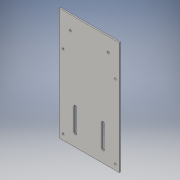
# Autodesk Inventor part: Part2
Saved by Autodesk Inventor 2016 (Build 200138000, 138)
## iProperties
Created: 2015-10-15
Part Number: Part2
Material: Generic
Document SubType Name: Modeling
Designer: hozhu
Density: 1 g/cm^3
Appearance: Default
Author: hozhu
Autodesk Inventor part; units mm, degrees
ref_plane "YZ Plane" through (0, 0, 0) normal (1, 0, 0) x (0, 1, 0)
ref_plane "XZ Plane" through (0, 0, 0) normal (0, 1, 0) x (-1, 0, 0)
ref_plane "XY Plane" through (0, 0, 0) normal (0, 0, 1) x (1, 0, 0)
sketch "Sketch1" plane through (0, 0, 0) normal (0, 0, 1) x (1, 0, 0)
  line L0 (-68.58, -128.7145) -> (68.58, -128.7145)
  line L1 (68.58, -128.7145) -> (68.58, 128.7145)
  line L2 (68.58, 128.7145) -> (-68.58, 128.7145)
  line L3 (-68.58, 128.7145) -> (-68.58, -128.7145)
  line L4 (-68.58, -128.7145) -> (68.58, 128.7145) construction
  line L5 (68.58, -128.7145) -> (-68.58, 128.7145) construction
  point P0 (0, 0)
  dimension "d0" = 137.16
  dimension "d1" = 257.429
  constraints: 12 end point, 2 midpoint, 2 parallel, 1 horizontal, 1 perpendicular
  measures "d0" distance of L1.end L2.end
  measures "d1" distance of L2.end L0.start
extrude "Extrusion1" add sketch "Sketch1" against normal blind 3.175
sketch "Sketch2" plane through (0, 0, 0) normal (0, 0, 1) x (1, 0, 0)
  circle A0 centre (-59.69, 52.5145) radius 2.0955
  line L0 (-68.58, 128.7145) -> (-68.58, -128.7145) projected
  line L1 (-68.58, 128.7145) -> (68.58, 128.7145) projected
  circle A1 centre (59.69, 52.5145) radius 2.0955
  line L2 (68.58, -128.7145) -> (68.58, 128.7145) projected
  circle A2 centre (-59.69, -116.0145) radius 2.0955
  circle A3 centre (59.69, -116.0145) radius 2.0955
  line L3 (-68.58, -128.7145) -> (68.58, -128.7145) projected
  point P0 (0, 0)
  dimension "d4" = 8.89
  dimension "d5" = 76.2
  dimension "d6" = 76.2
  dimension "d7" = 8.89
  dimension "d8" = 4.191
  dimension "d9" = 12.7
  dimension "d10" = 8.89
  dimension "d11" = 8.89
  dimension "d12" = 12.7
  dimension "d13" = 4.191
  dimension "d21" = 4.191
  dimension "d22" = 4.191
  constraints: 4 centre point
  measures "d4" distance from line of L0 A0.centre
  measures "d5" distance from line of L1 A0.centre
  measures "d6" distance from line of L1 A1.centre
  measures "d7" distance from line of A1.centre L2
  measures "d8" diameter of A1
  measures "d9" distance from line of L3 A2.centre
  measures "d10" distance from line of L0 A2.centre
  measures "d11" distance from line of L2 A3.centre
  measures "d12" distance from line of L3 A3.centre
  measures "d13" diameter of A0
  measures "d21" diameter of A2
  measures "d22" diameter of A3
hole "Hole1" at (-59.69, 52.5145, 0) at (59.69, 52.5145, 0) at (-59.69, -116.0145, 0) at (59.69, -116.0145, 0) direction (0, 0, -1) diameter 4.191 end through all
sketch "Sketch4" plane through (0, 0, 0) normal (0, 0, 1) x (1, 0, 0)
  line L0 (-35.179, -49.0855) -> (-35.179, -99.8855)
  line L1 (-28.321, -49.0855) -> (-28.321, -99.8855)
  line L2 (28.321, -49.0855) -> (28.321, -99.8855)
  line L3 (35.179, -49.0855) -> (35.179, -99.8855)
  line L4 (-68.58, 128.7145) -> (-68.58, -128.7145) projected
  line L5 (68.58, -128.7145) -> (68.58, 128.7145) projected
  line L6 (-68.58, -128.7145) -> (68.58, -128.7145) projected
  arc A0 (-28.321, -49.0855) -> (-35.179, -49.0855) centre (-31.75, -49.0855) ccw
  arc A1 (-35.179, -99.8855) -> (-28.321, -99.8855) centre (-31.75, -99.8855) ccw
  arc A2 (35.179, -49.0855) -> (28.321, -49.0855) centre (31.75, -49.0855) ccw
  arc A3 (28.321, -99.8855) -> (35.179, -99.8855) centre (31.75, -99.8855) ccw
  point P0 (0, 0)
  dimension "d23" = 6.858
  dimension "d24" = 6.858
  dimension "d25" = 33.401
  dimension "d26" = 50.8
  dimension "d27" = 33.401
  dimension "d28" = 28.829
  dimension "d29" = 28.829
  dimension "d30" = 28.829
  dimension "d31" = 28.829
  dimension "d32" = 50.8
  dimension "d33" = 50.8
  dimension "d34" = 50.8
  constraints: 8 end point, 8 point on circle, 4 centre point, 4 tangent, 4 vertical
  measures "d23" distance of L1.end L0.end
  measures "d24" distance between parallel lines of L3 L2
  measures "d25" distance between parallel lines of L4 L0
  measures "d26" distance of L3.start L3.end
  measures "d27" distance between parallel lines of L5 L3
  measures "d28" distance from line of L6 L0.end
  measures "d29" distance from line of L6 L1.end
  measures "d30" distance from line of L6 L2.end
  measures "d31" distance from line of L6 L3.end
  measures "d32" distance of L0.start L0.end
  measures "d33" distance of L1.start L1.end
  measures "d34" distance of L2.start L2.end
extrude "Extrusion2" cut sketch "Sketch4" against normal blind 3.175
sketch "Sketch5" plane through (0, 0, 0) normal (0, 0, 1) x (1, 0, 0)
  line L0 (-68.58, 128.7145) -> (68.58, 128.7145) projected
  line L1 (68.58, 128.7145) -> (68.58, -128.7145) projected
  point P0 (0, 0)
  point P1 (-43.3324, 96.9645)
  point P2 (43.3324, 96.9645)
  dimension "d37" = 31.75
  dimension "d38" = 86.6648
  dimension "d39" = 31.75
  dimension "d40" = 25.2476
  measures "d37" distance from line of L0 point (-43.332, 96.964)
  measures "d38" distance of point (-43.332, 96.964) point (43.332, 96.964)
  measures "d39" distance from line of L0 point (43.332, 96.964)
  measures "d40" distance from line of L1 point (43.332, 96.964)
hole "Hole2" at (-43.3324, 96.9645, 0) at (43.3324, 96.9645, 0) direction (0, 0, -1) diameter 4.4704 end through all
sketch "battery_buzzer" plane through (0, 0, 0) normal (0, 0, 1) x (1, 0, 0)
  line L0 (-50.8, 39.8145) -> (50.8, 39.8145)
  line L1 (50.8, 39.8145) -> (50.8, -36.3855)
  line L2 (50.8, -36.3855) -> (-50.8, -36.3855)
  line L3 (-50.8, -36.3855) -> (-50.8, 39.8145)
  line L4 (68.58, -128.7145) -> (68.58, 128.7145) projected
  line L5 (68.58, 128.7145) -> (-68.58, 128.7145) projected
  line L6 (-68.58, 128.7145) -> (-68.58, -128.7145) projected
  line L7 (-44.45, 33.4645) -> (-11.43, 33.4645)
  line L8 (-11.43, 33.4645) -> (-11.43, 5.5245)
  line L9 (-11.43, 5.5245) -> (-44.45, 5.5245)
  line L10 (-44.45, 5.5245) -> (-44.45, 33.4645)
  circle A0 centre (-40.64, 29.6545) radius 1.651
  circle A1 centre (-40.64, 8.6995) radius 1.651
  circle A2 centre (-15.24, 8.6995) radius 1.651
  line L11 (0.508, 33.4645) -> (33.528, 33.4645)
  line L12 (33.528, 33.4645) -> (33.528, 5.5245)
  line L13 (33.528, 5.5245) -> (0.508, 5.5245)
  line L14 (0.508, 5.5245) -> (0.508, 33.4645)
  circle A3 centre (4.318, 29.6545) radius 1.651
  circle A4 centre (4.318, 8.6995) radius 1.651
  circle A5 centre (29.718, 8.6995) radius 1.651
  line L15 (-44.45, 1.7145) -> (-11.43, 1.7145)
  line L16 (-11.43, 1.7145) -> (-11.43, -26.2255)
  line L17 (-11.43, -26.2255) -> (-44.45, -26.2255)
  line L18 (-44.45, -26.2255) -> (-44.45, 1.7145)
  circle A6 centre (-40.64, -2.0955) radius 1.651
  circle A7 centre (-40.64, -23.0505) radius 1.651
  circle A8 centre (-15.2413, -22.7965) radius 1.651
  line L19 (33.5293, 1.9685) -> (33.5293, -27.2717)
  circle A9 centre (29.718, -23.0505) radius 1.651
  line L20 (33.5293, -27.2717) -> (0.5093, -27.2717)
  line L21 (0.5093, 1.9685) -> (33.5293, 1.9685)
  circle A10 centre (4.3193, -22.7965) radius 1.651
  circle A11 centre (4.3193, -1.8415) radius 1.651
  line L22 (0.5093, -27.2717) -> (0.5093, 1.9685)
  point P0 (-1.6153, -4.4833)
  point P1 (48.3688, -4.4833)
  dimension "d48" = 17.78
  dimension "d49" = 88.9
  dimension "d50" = 76.2
  dimension "d51" = 17.78
  dimension "d52" = 33.02
  dimension "d54" = 3.302
  dimension "d55" = 3.302
  dimension "d57" = 3.81
  dimension "d58" = 3.81
  dimension "d59" = 3.81
  dimension "d60" = 20.955
  dimension "d62" = 25.4
  dimension "d74" = 33.02
  dimension "d75" = 3.302
  dimension "d76" = 3.302
  dimension "d77" = 3.81
  dimension "d78" = 3.81
  dimension "d79" = 3.81
  dimension "d80" = 20.955
  dimension "d81" = 25.4
  dimension "d183" = 6.35
  dimension "d184" = 6.35
  dimension "d185" = 6.35
  dimension "d186" = 27.94
  dimension "d205" = 80.518
  dimension "d206" = 33.02
  dimension "d207" = 3.302
  dimension "d208" = 3.302
  dimension "d209" = 3.81
  dimension "d210" = 3.81
  dimension "d211" = 3.81
  dimension "d212" = 20.955
  dimension "d213" = 25.4
  dimension "d214" = 33.02
  dimension "d215" = 3.302
  dimension "d216" = 3.302
  dimension "d217" = 3.81
  dimension "d218" = 3.81
  dimension "d219" = 3.81
  dimension "d220" = 20.955
  dimension "d221" = 25.4
  dimension "d222" = 27.94
  dimension "d223" = 41.656
  dimension "d225" = 80.518
  dimension "d227" = 6.35
  dimension "d230" = 62.865
  dimension "d231" = 62.865
  constraints: 40 end point, 13 perpendicular, 12 centre point, 5 horizontal, 2 parallel
  measures "d48" distance between parallel lines of L4 L1
  measures "d49" distance between parallel lines of L5 L0
  measures "d50" distance of L0.end L1.end
  measures "d51" distance between parallel lines of L6 L3
  measures "d52" distance of L7.start L7.end
  measures "d54" diameter of A0
  measures "d55" diameter of A1
  measures "d57" distance from line of L7 A0.centre
  measures "d58" distance from line of L10 A1.centre
  measures "d59" distance from line of L10 A0.centre
  measures "d60" distance of A1.centre A0.centre
  measures "d62" distance of A1.centre A2.centre
  measures "d74" distance of L11.start L12.start
  measures "d75" diameter of A3
  measures "d76" diameter of A4
  measures "d77" distance from line of L11 A3.centre
  measures "d78" distance from line of L14 A4.centre
  measures "d79" distance from line of L14 A3.centre
  measures "d80" distance of A4.centre A3.centre
  measures "d81" distance of A4.centre A5.centre
  measures "d183" distance between parallel lines of L3 L10
  measures "d184" distance between parallel lines of L0 L7
  measures "d185" distance between parallel lines of L0 L11
  measures "d186" distance of L7.end L8.end
  measures "d205" distance from line of L3 A5.centre
  measures "d206" distance of L15.start L15.end
  measures "d207" diameter of A6
  measures "d208" diameter of A7
  measures "d209" distance from line of L15 A6.centre
  measures "d210" distance from line of L18 A7.centre
  measures "d211" distance from line of L18 A6.centre
  measures "d212" distance of A7.centre A6.centre
  measures "d213" distance of A7.centre A8.centre
  measures "d214" distance of L21.start L19.start
  measures "d215" diameter of A11
  measures "d216" diameter of A10
  measures "d217" distance from line of L21 A11.centre
  measures "d218" distance from line of L22 A10.centre
  measures "d219" distance from line of L22 A11.centre
  measures "d220" distance of A10.centre A11.centre
  measures "d221" distance of A10.centre A9.centre
  measures "d222" distance of L15.end L17.start
  measures "d223" distance from line of L0 A11.centre
  measures "d225" distance from line of L3 A9.centre
  measures "d227" distance between parallel lines of L3 L18
  measures "d230" distance from line of A7.centre L0
  measures "d231" distance from line of L0 A9.centre
sketch "grizzly_bear" plane through (0, 0, 0) normal (0, 0, 1) x (1, 0, 0)
  line L0 (-50.8, 39.8145) -> (50.8, 39.8145)
  line L1 (50.8, 39.8145) -> (50.8, -36.3855)
  line L2 (50.8, -36.3855) -> (-50.8, -36.3855)
  line L3 (-50.8, -36.3855) -> (-50.8, 39.8145)
  line L4 (-68.58, 128.7145) -> (-68.58, -128.7145) projected
  line L5 (68.58, -128.7145) -> (68.58, 128.7145) projected
  line L6 (68.58, 128.7145) -> (-68.58, 128.7145) projected
  line L7 (-43.688, -8.4455) -> (32.512, -8.4455)
  line L8 (32.512, -8.4455) -> (32.512, 32.8295)
  line L9 (32.512, 32.8295) -> (-43.688, 32.8295)
  line L10 (-43.688, 32.8295) -> (-43.688, -8.4455)
  circle A0 centre (-40.64, 29.6545) radius 1.651
  circle A1 centre (29.718, -5.6515) radius 1.651
  circle A2 centre (29.718, 29.6545) radius 1.651
  circle A3 centre (21.123, -3.4255) radius 0.45
  circle A4 centre (16.723, -3.4255) radius 0.45
  dimension "d100" = 17.78
  dimension "d101" = 17.78
  dimension "d102" = 88.9
  dimension "d103" = 76.2
  dimension "d187" = 3.302
  dimension "d188" = 0.9
  dimension "d189" = 76.2
  dimension "d190" = 41.275
  dimension "d191" = 2.794
  dimension "d192" = 3.175
  dimension "d193" = 38.481
  dimension "d194" = 73.406
  dimension "d195" = 11.389
  dimension "d196" = 36.255
  dimension "d197" = 15.789
  dimension "d198" = 36.255
  dimension "d199" = 73.152
  dimension "d200" = 3.175
  dimension "d203" = 10.16
  dimension "d204" = 10.16
  constraints: 16 end point, 5 centre point, 3 equal radius, 3 parallel, 3 perpendicular, 1 horizontal
  measures "d100" distance between parallel lines of L4 L3
  measures "d101" distance between parallel lines of L5 L1
  measures "d102" distance between parallel lines of L6 L0
  measures "d103" distance of L0.end L1.end
  measures "d187" diameter of A2
  measures "d188" diameter of A3
  measures "d189" distance between parallel lines of L8 L10
  measures "d190" distance between parallel lines of L7 L9
  measures "d191" distance from line of A2.centre L8
  measures "d192" distance from line of A2.centre L9
  measures "d193" distance from line of A1.centre L9
  measures "d194" distance from line of A1.centre L10
  measures "d195" distance from line of A3.centre L8
  measures "d196" distance from line of A3.centre L9
  measures "d197" distance from line of A4.centre L8
  measures "d198" distance from line of A4.centre L9
  measures "d199" distance from line of A0.centre L8
  measures "d200" distance from line of A0.centre L9
  measures "d203" distance from line of L0 A0.centre
  measures "d204" distance from line of L3 A0.centre
sketch "Smartsensor" plane through (0, 0, 0) normal (0, 0, 1) x (1, 0, 0)
  line L0 (-34.6866, -23.8471) -> (-34.6866, 4.0929)
  line L1 (-34.6866, 4.0929) -> (-1.6666, 4.0929)
  line L2 (-1.6666, 4.0929) -> (-1.6666, -23.8471)
  line L3 (-34.6866, -23.8471) -> (-1.6666, -23.8471)
  circle A0 centre (-30.8766, 0.2829) radius 1.651
  circle A1 centre (-5.4766, -20.6721) radius 1.651
  circle A2 centre (-4.2066, -16.2271) radius 1
  circle A3 centre (-4.2066, -13.6871) radius 1
  circle A4 centre (-4.2066, -11.1471) radius 1
  circle A5 centre (-4.2066, -8.6071) radius 1
  circle A6 centre (-4.2066, -6.0671) radius 1
  circle A7 centre (-4.2066, -3.5271) radius 1
  line L4 (0.8734, -23.8471) -> (0.8734, 4.0929)
  line L5 (0.8734, 4.0929) -> (33.8934, 4.0929)
  line L6 (33.8934, 4.0929) -> (33.8934, -23.8471)
  line L7 (0.8734, -23.8471) -> (33.8934, -23.8471)
  circle A8 centre (4.6834, 0.2829) radius 1.651
  circle A9 centre (30.0834, -20.6721) radius 1.651
  circle A10 centre (31.3534, -16.2271) radius 1
  circle A11 centre (31.3534, -13.6871) radius 1
  circle A12 centre (31.3534, -11.1471) radius 1
  circle A13 centre (31.3534, -8.6071) radius 1
  circle A14 centre (31.3534, -6.0671) radius 1
  circle A15 centre (31.3534, -3.5271) radius 1
  line L8 (-50.8, 39.8145) -> (50.8, 39.8145)
  line L9 (50.8, 39.8145) -> (50.8, -36.3855)
  line L10 (50.8, -36.3855) -> (-50.8, -36.3855)
  line L11 (-50.8, -36.3855) -> (-50.8, 39.8145)
  line L12 (68.58, -128.7145) -> (68.58, 128.7145) projected
  line L13 (-68.58, 128.7145) -> (-68.58, -128.7145) projected
  line L14 (68.58, 128.7145) -> (-68.58, 128.7145) projected
  point P0 (0, 0)
  dimension "d104" = 17.78
  dimension "d105" = 17.78
  dimension "d106" = 88.9
  dimension "d107" = 76.2
  constraints: 24 end point, 16 centre point, 2 parallel, 1 horizontal, 1 perpendicular
  measures "d104" distance between parallel lines of L12 L9
  measures "d105" distance between parallel lines of L13 L11
  measures "d106" distance between parallel lines of L14 L8
  measures "d107" distance of L10.end L8.start
sketch "SmartsensorPowered" plane through (0, 0, 0) normal (0, 0, 1) x (1, 0, 0)
  line L0 (-31.115, 32.8295) -> (-3.175, 32.8295)
  line L1 (-3.175, 32.8295) -> (-3.175, -26.8605)
  line L2 (-3.175, -26.8605) -> (-31.115, -26.8605)
  line L3 (-31.115, -26.8605) -> (-31.115, 32.8295)
  circle A0 centre (-27.94, 29.6545) radius 1.651
  circle A1 centre (-27.305, -23.0505) radius 1.651
  circle A2 centre (-6.35, 2.3495) radius 1.651
  circle A3 centre (-6.35, 29.6545) radius 1.651
  circle A4 centre (18.415, -23.0505) radius 1.651
  circle A5 centre (39.37, 2.3495) radius 1.651
  circle A6 centre (17.78, 29.6545) radius 1.651
  line L4 (14.605, -26.8605) -> (14.605, 32.8295)
  circle A7 centre (39.37, 29.6545) radius 1.651
  line L5 (14.605, 32.8295) -> (42.545, 32.8295)
  line L6 (42.545, 32.8295) -> (42.545, -26.8605)
  line L7 (42.545, -26.8605) -> (14.605, -26.8605)
  line L8 (-50.8, 39.8145) -> (50.8, 39.8145)
  line L9 (50.8, 39.8145) -> (50.8, -36.3855)
  line L10 (50.8, -36.3855) -> (-50.8, -36.3855)
  line L11 (-50.8, -36.3855) -> (-50.8, 39.8145)
  line L12 (-68.58, 128.7145) -> (-68.58, -128.7145) projected
  line L13 (68.58, 128.7145) -> (68.58, -128.7145) projected
  line L14 (68.58, 128.7145) -> (-68.58, 128.7145) projected
  point P0 (0, 0)
  dimension "d108" = 27.94
  dimension "d109" = 59.69
  dimension "d110" = 3.175
  dimension "d111" = 3.175
  dimension "d112" = 3.302
  dimension "d113" = 3.302
  dimension "d114" = 3.175
  dimension "d115" = 3.175
  dimension "d116" = 3.81
  dimension "d117" = 3.81
  dimension "d118" = 3.302
  dimension "d119" = 30.48
  dimension "d120" = 3.175
  dimension "d121" = 3.302
  dimension "d122" = 27.94
  dimension "d123" = 59.69
  dimension "d124" = 3.175
  dimension "d125" = 3.175
  dimension "d126" = 3.302
  dimension "d127" = 3.302
  dimension "d128" = 3.175
  dimension "d129" = 3.175
  dimension "d130" = 3.81
  dimension "d131" = 3.81
  dimension "d132" = 3.302
  dimension "d133" = 30.48
  dimension "d134" = 3.175
  dimension "d135" = 3.302
  dimension "d136" = 17.78
  dimension "d137" = 17.78
  dimension "d138" = 17.78
  dimension "d139" = 88.9
  dimension "d140" = 76.2
  dimension "d228" = 10.16
  dimension "d229" = 22.86
  constraints: 24 end point, 8 centre point, 6 parallel, 3 horizontal, 3 perpendicular, 1 collinear
  measures "d108" distance of L0.start L0.end
  measures "d109" distance of L2.end L0.start
  measures "d110" distance from line of L3 A0.centre
  measures "d111" distance from line of A0.centre L0
  measures "d112" diameter of A0
  measures "d113" diameter of A3
  measures "d114" distance from line of L1 A3.centre
  measures "d115" distance from line of L0 A3.centre
  measures "d116" distance from line of L2 A1.centre
  measures "d117" distance from line of L3 A1.centre
  measures "d118" diameter of A1
  measures "d119" distance from line of L0 A2.centre
  measures "d120" distance from line of L1 A2.centre
  measures "d121" diameter of A2
  measures "d122" distance of L4.end L5.end
  measures "d123" distance of L4.start L4.end
  measures "d124" distance from line of L4 A6.centre
  measures "d125" distance from line of A6.centre L5
  measures "d126" diameter of A6
  measures "d127" diameter of A7
  measures "d128" distance from line of L6 A7.centre
  measures "d129" distance from line of L5 A7.centre
  measures "d130" distance from line of L7 A4.centre
  measures "d131" distance from line of L4 A4.centre
  measures "d132" diameter of A4
  measures "d133" distance from line of L5 A5.centre
  measures "d134" distance from line of L6 A5.centre
  measures "d135" diameter of A5
  measures "d136" distance between parallel lines of L4 L1
  measures "d137" distance between parallel lines of L11 L12
  measures "d138" distance between parallel lines of L13 L9
  measures "d139" distance between parallel lines of L14 L8
  measures "d140" distance of L8.end L9.end
  measures "d228" distance from line of L8 A3.centre
  measures "d229" distance from line of L11 A0.centre
sketch "Teamflag" plane through (0, 0, 0) normal (0, 0, 1) x (1, 0, 0)
  line L0 (-3.81, -7.1755) -> (-44.45, -7.1755)
  line L1 (-44.45, -7.1755) -> (-44.45, 33.4645)
  line L2 (-44.45, 33.4645) -> (-3.81, 33.4645)
  line L3 (-3.81, 33.4645) -> (-3.81, -7.1755)
  circle A0 centre (-6.35, 30.9245) radius 1.651
  circle A1 centre (-41.91, 30.9245) radius 1.651
  circle A2 centre (-41.91, -4.6355) radius 1.651
  circle A3 centre (-6.35, -4.6355) radius 1.651
  line L4 (43.18, -7.1755) -> (2.54, -7.1755)
  circle A4 centre (5.08, -4.6355) radius 1.651
  circle A5 centre (40.64, -4.6355) radius 1.651
  line L5 (2.54, -7.1755) -> (2.54, 33.4645)
  line L6 (43.18, 33.4645) -> (43.18, -7.1755)
  circle A6 centre (40.64, 30.9245) radius 1.651
  line L7 (2.54, 33.4645) -> (43.18, 33.4645)
  circle A7 centre (5.08, 30.9245) radius 1.651
  line L8 (-50.8, 39.8145) -> (50.8, 39.8145)
  line L9 (50.8, 39.8145) -> (50.8, -36.3855)
  line L10 (50.8, -36.3855) -> (-50.8, -36.3855)
  line L11 (-50.8, -36.3855) -> (-50.8, 39.8145)
  line L12 (68.58, 128.7145) -> (68.58, -128.7145) projected
  line L13 (-68.58, -128.7145) -> (-68.58, 128.7145) projected
  line L14 (-68.58, 128.7145) -> (68.58, 128.7145) projected
  point P0 (0, 0)
  dimension "d141" = 3.302
  dimension "d142" = 40.64
  dimension "d143" = 40.64
  dimension "d144" = 2.54
  dimension "d145" = 2.54
  dimension "d146" = 2.54
  dimension "d147" = 38.1
  dimension "d148" = 38.1
  dimension "d149" = 2.54
  dimension "d150" = 38.1
  dimension "d151" = 38.1
  dimension "d152" = 3.302
  dimension "d153" = 40.64
  dimension "d154" = 40.64
  dimension "d155" = 2.54
  dimension "d156" = 2.54
  dimension "d157" = 2.54
  dimension "d158" = 38.1
  dimension "d159" = 38.1
  dimension "d160" = 2.54
  dimension "d161" = 38.1
  dimension "d162" = 38.1
  dimension "d163" = 6.35
  dimension "d164" = 17.78
  dimension "d165" = 17.78
  dimension "d166" = 88.9
  dimension "d167" = 76.2
  constraints: 24 end point, 8 centre point, 6 equal radius, 6 parallel, 3 horizontal, 2 vertical, 1 collinear, 1 perpendicular
  measures "d141" diameter of A0
  measures "d142" distance between parallel lines of L1 L3
  measures "d143" distance between parallel lines of L2 L0
  measures "d144" distance from line of A0.centre L3
  measures "d145" distance from line of A0.centre L2
  measures "d146" distance from line of A3.centre L3
  measures "d147" distance from line of A3.centre L2
  measures "d148" distance from line of A1.centre L3
  measures "d149" distance from line of A1.centre L2
  measures "d150" distance from line of A2.centre L3
  measures "d151" distance from line of A2.centre L2
  measures "d152" diameter of A6
  measures "d153" distance between parallel lines of L5 L6
  measures "d154" distance between parallel lines of L7 L4
  measures "d155" distance from line of A6.centre L6
  measures "d156" distance from line of A6.centre L7
  measures "d157" distance from line of A5.centre L6
  measures "d158" distance from line of A5.centre L7
  measures "d159" distance from line of A7.centre L6
  measures "d160" distance from line of A7.centre L7
  measures "d161" distance from line of A4.centre L6
  measures "d162" distance from line of A4.centre L7
  measures "d163" distance between parallel lines of L5 L3
  measures "d164" distance between parallel lines of L12 L9
  measures "d165" distance between parallel lines of L13 L11
  measures "d166" distance between parallel lines of L14 L8
  measures "d167" distance of L8.end L9.end
sketch "Cape" plane through (0, 0, 0) normal (0, 0, 1) x (1, 0, 0)
  line L0 (-44.45, -21.1355) -> (27.61, -21.1355)
  line L1 (27.61, -21.1355) -> (27.61, 33.4645)
  line L2 (27.61, 33.4645) -> (-44.45, 33.4645)
  line L3 (-44.45, 33.4645) -> (-44.45, -21.1355)
  circle A0 centre (-41.275, -17.9605) radius 1.5875
  circle A1 centre (24.765, -14.7855) radius 1.5875
  circle A2 centre (24.765, 27.1245) radius 1.5875
  circle A3 centre (-41.275, 30.2995) radius 1.5875
  line L4 (-50.8, 39.8145) -> (50.8, 39.8145)
  line L5 (50.8, 39.8145) -> (50.8, -36.3855)
  line L6 (50.8, -36.3855) -> (-50.8, -36.3855)
  line L7 (-50.8, -36.3855) -> (-50.8, 39.8145)
  line L8 (68.58, -128.7145) -> (68.58, 128.7145) projected
  line L9 (-68.58, 128.7145) -> (-68.58, -128.7145) projected
  line L10 (68.58, 128.7145) -> (-68.58, 128.7145) projected
  point P0 (0, 0)
  point P1 (0, 0)
  dimension "d168" = 3.175
  dimension "d169" = 72.06
  dimension "d170" = 54.6
  dimension "d171" = 2.845
  dimension "d172" = 6.34
  dimension "d173" = 2.845
  dimension "d174" = 48.25
  dimension "d175" = 68.885
  dimension "d176" = 3.165
  dimension "d177" = 68.885
  dimension "d178" = 51.425
  dimension "d179" = 17.78
  dimension "d180" = 17.78
  dimension "d181" = 88.9
  dimension "d182" = 76.2
  constraints: 16 end point, 4 centre point, 4 parallel, 3 equal radius, 2 horizontal, 1 perpendicular, 1 vertical
  measures "d168" diameter of A2
  measures "d169" distance between parallel lines of L1 L3
  measures "d170" distance between parallel lines of L2 L0
  measures "d171" distance from line of A2.centre L1
  measures "d172" distance from line of A2.centre L2
  measures "d173" distance from line of A1.centre L1
  measures "d174" distance from line of A1.centre L2
  measures "d175" distance from line of A3.centre L1
  measures "d176" distance from line of A3.centre L2
  measures "d177" distance from line of A0.centre L1
  measures "d178" distance from line of A0.centre L2
  measures "d179" distance between parallel lines of L8 L5
  measures "d180" distance between parallel lines of L9 L7
  measures "d181" distance between parallel lines of L10 L4
  measures "d182" distance of L4.end L5.end
body "Solid1"
